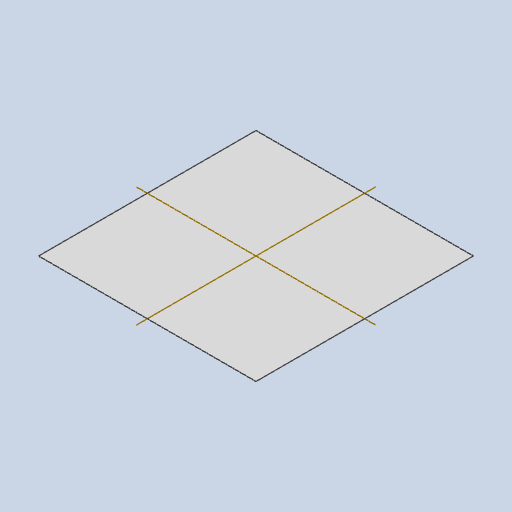
# Autodesk Inventor part: Ground
Saved by Autodesk Inventor 2023 (Build 270158000, 158)
## iProperties
Created: 2023-01-12
Part Number: Ground
Material: Generic
Document SubType Name: Modeling
Designer: rosam
Density: 1 g/cm^3
Appearance: Default
Author: rosam
Autodesk Inventor part; units mm, degrees
ref_plane "YZ Plane" through (0, 0, 0) normal (1, 0, 0) x (0, 1, 0)
ref_plane "XZ Plane" through (0, 0, 0) normal (0, 1, 0) x (-1, 0, 0)
ref_plane "XY Plane" through (0, 0, 0) normal (0, 0, 1) x (1, 0, 0)
sketch "Sketch1" plane through (0, 0, 0) normal (0, 1, 0) x (-1, 0, 0)
  line L0 (1270, 1270) -> (-1270, 1270)
  line L1 (-1270, 1270) -> (-1270, -1270)
  line L2 (-1270, -1270) -> (1270, -1270)
  line L3 (1270, -1270) -> (1270, 1270)
  point P0 (0, 0)
  dimension "d2" = 1270
  dimension "d3" = 1270
  dimension "d4" = 2540
  constraints: 8 end point, 2 parallel, 2 perpendicular, 1 horizontal
  measures "d2" distance from line of point (0, 0) L0
  measures "d3" distance from line of point (0, 0) L1
  measures "d4" distance of L1.end L2.end
extrude "Extrusion1" add sketch "Sketch1" along normal blind 2.54
ref_plane "Work Plane1" through (-1270, 0, 0) normal (0, 0, 1) x (1, 0, 0)
ref_plane "Work Plane2" through (0, 0, 1270) normal (1, 0, 0) x (0, 0, -1)
equation "\"d2\" = 0.5 * d4"
equation "\"d3\" = 0.5 * d4"
body "Solid1"
